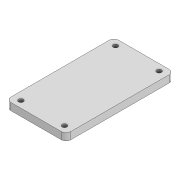
# Autodesk Inventor part: Plastic base
Saved by Autodesk Inventor 2020 (Build 240168000, 168)
## iProperties
Created: 2021-03-15
Part Number: Plastic base
Material: Generic
Document SubType Name: Modeling
Designer: ferrerx
Density: 1 g/cm^3
Appearance: Default
Author: ferrerx
Autodesk Inventor part; units mm, degrees
ref_plane "YZ Plane" through (0, 0, 0) normal (1, 0, 0) x (0, 1, 0)
ref_plane "XZ Plane" through (0, 0, 0) normal (0, 1, 0) x (-1, 0, 0)
ref_plane "XY Plane" through (0, 0, 0) normal (0, 0, 1) x (1, 0, 0)
sketch "Sketch1" plane through (0, 0, 0) normal (0, 1, 0) x (-1, 0, 0)
  line L0 (-9.1, 19.75) -> (9.1, 19.75) construction
  line L1 (9.1, 19.75) -> (9.1, -19.75) construction
  line L2 (9.1, -19.75) -> (-9.1, -19.75) construction
  line L3 (-9.1, -19.75) -> (-9.1, 19.75) construction
  line L4 (-9.1, 19.75) -> (9.1, -19.75) construction
  line L5 (9.1, 19.75) -> (-9.1, -19.75) construction
  line L6 (-12.5, 22.5) -> (12.5, 22.5)
  line L7 (12.5, 22.5) -> (12.5, -22.5)
  line L8 (12.5, -22.5) -> (-12.5, -22.5)
  line L9 (-12.5, -22.5) -> (-12.5, 22.5)
  line L10 (-12.5, 22.5) -> (12.5, -22.5) construction
  line L11 (12.5, 22.5) -> (-12.5, -22.5) construction
  circle A0 centre (9.1, 19.75) radius 1
  circle A1 centre (9.1, -19.75) radius 1
  circle A2 centre (-9.1, -19.75) radius 1
  circle A3 centre (-9.1, 19.75) radius 1
  point P0 (0, 0)
  dimension "d0" = 39.5
  dimension "d1" = 18.2
  dimension "d2" = 2
  dimension "d3" = 2
  dimension "d4" = 2
  dimension "d5" = 2
  dimension "d6" = 45
  dimension "d7" = 25
  constraints: 24 end point, 4 centre point, 4 coincident, 4 midpoint, 4 parallel, 2 horizontal, 2 perpendicular
  measures "d0" distance of L0.end L1.end
  measures "d1" distance of L1.end L2.end
  measures "d2" diameter of A0
  measures "d3" diameter of A3
  measures "d4" diameter of A2
  measures "d5" diameter of A1
  measures "d6" distance of L6.end L7.end
  measures "d7" distance of L7.end L8.end
extrude "Extrusion1" add sketch "Sketch1" along normal blind 3
fillet "Fillet1" radius 2 4 edges at (12.5, 1.5, -22.5) (-12.5, 1.5, -22.5) (12.5, 1.5, 22.5) (-12.5, 1.5, 22.5)
body "Solid1"
